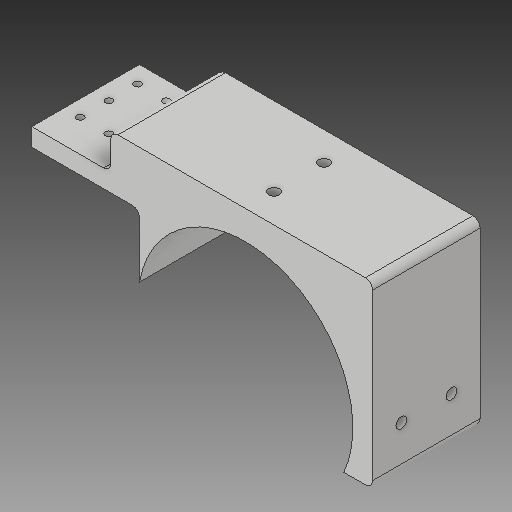
# Autodesk Inventor part: support-trappe
Saved by Autodesk Inventor 2017 (Build 210142000, 142)
## iProperties
Created: 2018-04-01
Part Number: support-trappe
Material: Generic
Document SubType Name: Modeling
Designer: franc
Density: 1 g/cm^3
Appearance: Default
Mass: 40.5741 g
Surface Area: 124.996 cm^2
Volume: 40.5741 cm^3
Author: franc
Autodesk Inventor part; units mm, degrees
ref_plane "YZ Plane" through (0, 0, 0) normal (1, 0, 0) x (0, 1, 0)
ref_plane "XZ Plane" through (0, 0, 0) normal (0, 1, 0) x (-1, 0, 0)
ref_plane "XY Plane" through (0, 0, 0) normal (0, 0, 1) x (1, 0, 0)
sketch "Esquisse1" plane through (0, 0, 0) normal (0, 1, 0) x (-1, 0, 0)
  line L0 (11.9492, 16.7797) -> (-18.0508, 16.7797)
  line L1 (-18.0508, 16.7797) -> (-18.0508, -13.2203)
  line L2 (-18.0508, -13.2203) -> (11.9492, -13.2203)
  line L3 (11.9492, -13.2203) -> (11.9492, 16.7797)
  point P0 (0, 0)
  dimension "d0" = 30
  dimension "d1" = 30
  constraints: 8 end point, 2 parallel, 1 horizontal, 1 perpendicular
  measures "d0" distance of L2.end L0.start
  measures "d1" distance of L0.start L0.end
extrude "Extrusion1" add sketch "Esquisse1" along normal blind 5
sketch "Esquisse2" plane through (0, 5, 0) normal (0, 1, 0) x (1, 0, 0)
  line L0 (-11.9492, 17.2203) -> (-2.9492, 17.2203) projected
  line L1 (-11.9492, -16.7797) -> (-11.9492, 17.2203) projected
  line L2 (-11.9492, -16.7797) -> (-2.9492, -16.7797) projected
  line L3 (-2.9492, -15.7797) -> (-2.9492, -16.7797) projected
  line L4 (-2.9492, -15.7797) -> (5.0508, -15.7797) projected
  line L5 (5.0508, -15.7797) -> (5.0508, -16.7797) projected
  line L6 (5.0508, -16.7797) -> (13.0508, -16.7797) projected
  line L7 (13.0508, 17.2203) -> (13.0508, -16.7797) projected
  line L8 (5.0508, 17.2203) -> (13.0508, 17.2203) projected
  line L9 (5.0508, 16.2203) -> (5.0508, 17.2203) projected
  line L10 (-2.9492, 16.2203) -> (5.0508, 16.2203) projected
  line L11 (-2.9492, 16.2203) -> (-2.9492, 17.2203) projected
  circle A0 centre (-7.4492, 0.2203) radius 1 projected
  circle A1 centre (-7.4492, 8.2203) radius 1 projected
  circle A2 centre (-7.4492, -7.7797) radius 1 projected
  circle A3 centre (0.5508, -7.7797) radius 1 projected
  circle A4 centre (8.5508, 0.2203) radius 1 projected
  circle A5 centre (8.5508, 8.2203) radius 1 projected
  circle A6 centre (8.5508, -7.7797) radius 1 projected
  circle A7 centre (0.5508, 8.2203) radius 1 projected
  arc A8 (3.5508, -2.4254) -> (3.5508, 2.8661) centre (0.5508, 0.2203) ccw projected
  line L12 (3.5508, -2.4254) -> (3.5508, -4.7797) projected
  line L13 (3.5508, -4.7797) -> (-2.4492, -4.7797) projected
  line L14 (-2.4492, -4.7797) -> (-2.4492, -2.4254) projected
  arc A9 (-2.4492, 2.8661) -> (-2.4492, -2.4254) centre (0.5508, 0.2203) ccw projected
  line L15 (-2.4492, 2.8661) -> (-2.4492, 5.2203) projected
  line L16 (-2.4492, 5.2203) -> (3.5508, 5.2203) projected
  line L17 (3.5508, 5.2203) -> (3.5508, 2.8661) projected
  circle A10 centre (8.5508, 8.2203) radius 1
  circle A11 centre (8.5508, 0.2203) radius 1
  circle A12 centre (8.5508, -7.7797) radius 1
  circle A13 centre (0.5508, -7.7797) radius 1
  circle A14 centre (-7.4492, -7.7797) radius 1
  circle A15 centre (-7.4492, 0.2203) radius 1
  circle A16 centre (-7.4492, 8.2203) radius 1
  circle A17 centre (0.5508, 8.2203) radius 1
  point P0 (0, 0)
  constraints: 8 centre point, 8 coincident, 8 concentric
extrude "Extrusion2" cut sketch "Esquisse2" against normal through all contours A0 | A1 | A2 | A3 | A4 | A5 | A6 | A7
sketch "Esquisse3" plane through (0, 5, 0) normal (0, 1, 0) x (1, 0, 0)
  line L0 (18.0508, 13.2203) -> (-11.9492, 13.2203) projected
  line L1 (10.0508, -16.7797) -> (10.0508, 13.2203)
  line L2 (-11.9492, -16.7797) -> (18.0508, -16.7797) projected
  line L3 (18.0508, -16.7797) -> (18.0508, 13.2203) projected
  line L4 (10.0508, 13.2203) -> (18.0508, 13.2203)
  line L5 (18.0508, 13.2203) -> (18.0508, -16.7797)
  line L6 (18.0508, -16.7797) -> (10.0508, -16.7797)
  line L7 (10.0508, -16.7797) -> (10.0508, 13.2203)
  point P0 (0, 0)
  dimension "d7" = 8
  constraints: 10 end point, 2 parallel, 1 horizontal, 1 perpendicular, 1 point on line
  measures "d7" distance between parallel lines of L3 L1
extrude "Extrusion3" add sketch "Esquisse3" along normal blind 10
fillet "Congé4" radius 2 1 edges at (10.0508, 5, 1.7797)
sketch "Esquisse5" plane through (-11.9492, 0, 16.7797) normal (0, 0, 1) x (1, 0, 0)
  circle A0 centre (59.5, -23) radius 30 projected
  line L0 (30, 0) -> (30, 15) projected
  line L1 (30, 15) -> (95, 15)
  line L2 (95, 15) -> (95, -35)
  line L3 (30, -17.5456) -> (30, 15)
  arc A1 (86.9955, -35) -> (30, -17.5456) centre (59.5, -23) ccw
  line L4 (95, -35) -> (86.9955, -35)
  line L5 (32.0045, -35) -> (30, -35)
  point P0 (11.9492, 0)
  dimension "d17" = 65
  dimension "d18" = 50
  constraints: 10 end point, 4 point on circle, 3 parallel, 1 centre point, 1 coincident, 1 concentric, 1 horizontal, 1 perpendicular
  measures "d17" distance of L0.end L1.end
  measures "d18" distance of L1.end L2.end
extrude "Extrusion4" add sketch "Esquisse5" against normal blind 30 contours A0 L3 L0 L1 L2 L4
fillet "Congé5" radius 2 1 edges at (18.0508, 0, 1.7797)
fillet "Congé6" radius 2 1 edges at (10.0508, 15, 1.7797)
fillet "Congé7" radius 2 1 edges at (83.0508, 15, 1.7797)
fillet "Congé8" radius 2 1 edges at (83.0508, -35, 1.7797)
sketch "Esquisse6" plane through (83.0508, 13, 16.7797) normal (1, 0, 0) x (0, 0, -1)
  circle A0 centre (8, -36) radius 1.5
  circle A1 centre (22, -36) radius 1.5
  line L0 (0, -46) -> (0, 0) projected
  line L1 (30, 0) -> (30, -46) projected
  line L2 (171, -6) -> (-4, -6)
  line L3 (171, -66) -> (-4, -66)
  point P0 (16.7797, -13)
  dimension "d25" = 3
  dimension "d26" = 3
  dimension "d27" = 8
  dimension "d28" = 8
  dimension "d29" = 30
  dimension "d30" = 30
  constraints: 4 end point, 2 centre point, 2 horizontal, 4 other
  measures "d25" diameter of A0
  measures "d26" diameter of A1
  measures "d27" distance from line of L0 A0.centre
  measures "d28" distance from line of L1 A1.centre
  measures "d29" distance from line of L2 A0.centre
  measures "d30" distance from line of L2 A1.centre
extrude "Extrusion5" cut sketch "Esquisse6" against normal through all
sketch "Esquisse7" plane through (0, 15, 0) normal (0, 1, 0) x (1, 0, 0)
  circle A0 centre (47.5508, 5.2203) radius 1.5
  circle A1 centre (47.5508, -8.7797) radius 1.5
  line L0 (12.0508, -16.7797) -> (81.0508, -16.7797) projected
  line L1 (12.0508, 13.2203) -> (81.0508, 13.2203) projected
  line L2 (17.5508, 154.2203) -> (17.5508, -20.7797)
  point P0 (0, 0)
  dimension "d33" = 3
  dimension "d34" = 3
  dimension "d35" = 8
  dimension "d36" = 8
  dimension "d37" = 30
  dimension "d38" = 30
  constraints: 2 centre point, 2 end point, 1 vertical, 2 other
  measures "d33" diameter of A0
  measures "d34" diameter of A1
  measures "d35" distance from line of L0 A1.centre
  measures "d36" distance from line of L1 A0.centre
  measures "d37" distance from line of L2 A0.centre
  measures "d38" distance from line of L2 A1.centre
extrude "Extrusion6" cut sketch "Esquisse7" against normal through all
